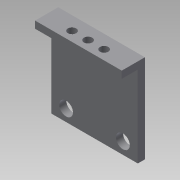
# Autodesk Inventor part: BodyToOpenCM
Saved by Autodesk Inventor 2014 (Build 180170000, 170)
## iProperties
Created: 2014-04-11
Part Number: BodyToOpenCM
Material: Générique
Document SubType Name: Modeling
Designer: Grégoire
Density: 1 g/cm^3
Appearance: Par défaut
Author: Grégoire
Autodesk Inventor part; units mm, degrees
ref_plane "YZ Plane" through (0, 0, 0) normal (1, 0, 0) x (0, 1, 0)
ref_plane "XZ Plane" through (0, 0, 0) normal (0, 1, 0) x (-1, 0, 0)
ref_plane "XY Plane" through (0, 0, 0) normal (0, 0, 1) x (1, 0, 0)
sketch "Esquisse1" plane through (0, 0, 0) normal (0, 1, 0) x (-1, 0, 0)
  line L0 (0, 0) -> (27, 0)
  line L1 (27, 0) -> (27, 27.55)
  line L2 (27, 27.55) -> (0, 27.55)
  line L3 (0, 27.55) -> (0, 0)
  circle A0 centre (4.65, 3.65) radius 2.15
  line L4 (13.5, 27.55) -> (13.5, 0) construction
  circle A1 centre (22.35, 3.65) radius 2.15
  dimension "d0" = 27
  dimension "d1" = 27.55
  dimension "d2" = 4.3
  dimension "d3" = 3.65
  dimension "d4" = 4.65
  constraints: 10 end point, 2 centre point, 2 midpoint, 2 parallel, 1 horizontal, 1 perpendicular, 1 symmetric about line, 1 other
  measures "d0" distance of L0.start L0.end
  measures "d1" distance of L2.end L0.start
  measures "d2" diameter of A0
  measures "d3" distance from line of L0 A0.centre
  measures "d4" distance from line of L3 A0.centre
extrude "Extrusion1" add sketch "Esquisse1" along normal blind 2.2
sketch "Esquisse2" plane through (0, 0, 0) normal (0, -1, 0) x (1, 0, 0)
  line L0 (0, 27.55) -> (0, 0) construction
  line L1 (-27, 27.55) -> (0, 27.55)
  line L2 (0, 27.55) -> (0, 25.35)
  line L3 (0, 25.35) -> (-27, 25.35)
  line L4 (-27, 25.35) -> (-27, 27.55)
  dimension "d7" = 2.2
  constraints: 8 end point, 2 parallel, 1 horizontal, 1 perpendicular, 1 point on line
  measures "d7" distance of L3.end L1.start
extrude "Extrusion2" add sketch "Esquisse2" along normal blind 5
sketch "Esquisse3" plane through (-27, 2.2, 27.55) normal (0, 0, 1) x (1, 0, 0)
  line L0 (27, -7.2) -> (27, 0) construction
  line L1 (0, -7.2) -> (0, 0) construction
  line L2 (27, -7.2) -> (0, -7.2) construction
  line L3 (0, -4.2) -> (27, -4.2) construction
  circle A0 centre (13.5, -4.2) radius 1.3
  circle A1 centre (18.5, -4.2) radius 1.3
  circle A2 centre (8.5, -4.2) radius 1.3
  circle A3 centre (13.5, -4.2) radius 1.3
  point P0 (27, -2.2)
  dimension "d10" = 3
  dimension "d11" = 2.6
  dimension "d14" = 5
  dimension "d17" = 5
  constraints: 4 centre point, 2 end point, 2 horizontal, 2 point on line, 1 midpoint, 1 perpendicular, 6 other
  measures "d10" distance between parallel lines of L2 L3
  measures "d11" diameter of A0
  measures "d14" distance of A0.centre A1.centre
  measures "d17" distance of A0.centre A2.centre
extrude "Extrusion3" cut sketch "Esquisse3" against normal through all
